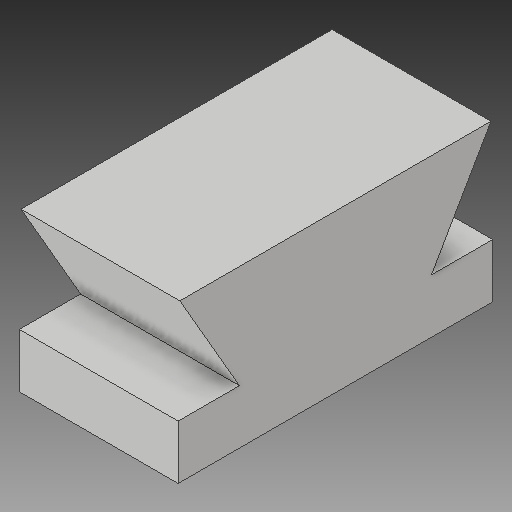
# Autodesk Inventor part: tester
Saved by Autodesk Inventor 2018 (Build 220112000, 112)
## iProperties
Created: 2018-09-13
Part Number: tester
Material: Generic
Document SubType Name: Modeling
Designer: David
Density: 1 g/cm^3
Appearance: Default
Author: David
Autodesk Inventor part; units mm, degrees
ref_plane "YZ Plane" through (0, 0, 0) normal (1, 0, 0) x (0, 1, 0)
ref_plane "XZ Plane" through (0, 0, 0) normal (0, 1, 0) x (-1, 0, 0)
ref_plane "XY Plane" through (0, 0, 0) normal (0, 0, 1) x (1, 0, 0)
sketch "Sketch1" plane through (0, 0, 0) normal (1, 0, 0) x (0, 1, 0)
  line L0 (-7.5, -12.5) -> (7.5, -12.5)
  line L1 (7.5, -12.5) -> (7.5, 12.5)
  line L2 (7.5, 12.5) -> (-7.5, 12.5)
  line L3 (-7.5, 12.5) -> (-7.5, -12.5)
  line L4 (-7.5, -12.5) -> (7.5, 12.5) construction
  line L5 (7.5, -12.5) -> (-7.5, 12.5) construction
  point P0 (0, 0)
  dimension "d0" = 25
  dimension "d1" = 15
  constraints: 12 end point, 2 midpoint, 2 parallel, 1 horizontal, 1 perpendicular
  measures "d0" distance of L0.end L1.end
  measures "d1" distance of L1.end L2.end
extrude "Extrusion1" add sketch "Sketch1" along normal blind 10
sketch "Sketch2" plane through (10, 0, 0) normal (1, 0, 0) x (0, 0, -1)
  line L0 (9.9, -7.5) -> (22, -7.5) projected
  line L1 (22, 12.5) -> (22, -7.5) projected
  line L2 (-35, 12.5) -> (22, 12.5) projected
  line L3 (-35, 12.5) -> (-35, 59.5) projected
  line L4 (-45, 59.5) -> (-35, 59.5) projected
  line L5 (-45, 59.5) -> (-45, -7.5) projected
  line L6 (-45, -7.5) -> (-9.9, -7.5) projected
  line L7 (-9.5, -7.5) -> (9.5, -7.5)
  line L8 (-9.9, -7.1) -> (-44.6, -7.1)
  line L9 (-44.6, -7.1) -> (-44.6, 59.1)
  line L10 (-44.6, 59.1) -> (-35.4, 59.1)
  line L11 (-35.4, 59.1) -> (-35.4, 12.1)
  line L12 (-35.4, 12.1) -> (21.6, 12.1)
  line L13 (21.6, 12.1) -> (21.6, -7.1)
  line L14 (21.6, -7.1) -> (9.9, -7.1)
  line L15 (9.9, -7.1) -> (9.9, -4.1)
  line L16 (9.9, -4.1) -> (6.04, -4.1)
  line L17 (6.04, -4.1) -> (9.7928, 2.4)
  line L18 (9.7928, 2.4) -> (-9.7928, 2.4)
  line L19 (-9.7928, 2.4) -> (-6.04, -4.1)
  line L20 (-6.04, -4.1) -> (-9.9, -4.1)
  line L21 (-9.9, -4.1) -> (-9.9, -7.1)
  line L22 (-9.9, -7.1) -> (-9.9, -7.5)
  line L23 (-12.5, -7.5) -> (12.5, -7.5) projected
  line L24 (9.9, -7.1) -> (9.9, -7.5)
  line L25 (-12.5, -7.5) -> (12.5, -7.5) projected
  circle A0 centre (-23.999, -0.85) radius 1.5 projected
  line L26 (-9.9, -7.5) -> (-9.9, -4.1) projected
  line L27 (-9.9, -4.1) -> (-6.04, -4.1) projected
  line L28 (-6.04, -4.1) -> (-9.7928, 2.4) projected
  line L29 (-9.7928, 2.4) -> (9.7928, 2.4) projected
  line L30 (9.7928, 2.4) -> (6.04, -4.1) projected
  line L31 (6.04, -4.1) -> (9.9, -4.1) projected
  line L32 (9.9, -4.1) -> (9.9, -7.5) projected
  point P0 (0, 0)
  constraints: 34 end point, 2 perpendicular, 2 point on line, 6 other
extrude "Extrusion2" cut sketch "Sketch2" against normal blind 10 contours L24 L14 L13 L12 L11 L10 L9 L8 L22 L6 L5 L4 L3 L2 L1 L0 | L15 L16 L17 L18 L19 L20 L21 L8 L9 L10 L11 L12 L13 L14 | A0
body "Solid1"
